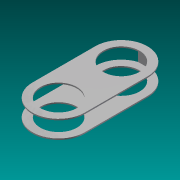
# Autodesk Inventor part: sambungan leaf spring 1
Saved by Autodesk Inventor 2014 SP2 (Build 180246200, 246)
## iProperties
Created: 2019-07-17
Part Number: sambungan leaf spring 1
Material: Steel, Mild
Document SubType Name: Modeling
Designer: USER PC
Density: 7.86 g/cm^3
Appearance: Steel
Author: USER PC
Autodesk Inventor part; units mm, degrees
ref_plane "YZ Plane" through (0, 0, 0) normal (1, 0, 0) x (0, 1, 0)
ref_plane "XZ Plane" through (0, 0, 0) normal (0, 1, 0) x (-1, 0, 0)
ref_plane "XY Plane" through (0, 0, 0) normal (0, 0, 1) x (1, 0, 0)
sketch "Sketch1" plane through (0, 0, 0) normal (0, 0, 1) x (1, 0, 0)
  circle A0 centre (0, 0) radius 35
  circle A1 centre (0, 120) radius 35
  arc A2 (-50, 0) -> (50, 0) centre (0, 0) ccw
  arc A3 (50, 120) -> (-50, 120) centre (0, 120) ccw
  line L0 (-50, 0) -> (-50, 120)
  line L1 (50, 0) -> (50, 120)
  line L2 (0, 35) -> (0, 85)
  dimension "d0" = 70
  dimension "d1" = 70
  dimension "d3" = 15
  dimension "d4" = 15
  dimension "d7" = 50
  constraints: 6 end point, 4 point on circle, 2 centre point, 2 tangent, 2 vertical alignment, 1 coincident, 1 parallel, 4 other
  measures "d7" distance of L2.start L2.end
extrude "Extrusion1" add sketch "Sketch1" along normal blind 35
sketch "Sketch2" plane through (50, 0, 0) normal (1, 0, 0) x (0, 0, -1)
  line L0 (-35, 170) -> (0, 170)
  line L1 (0, 170) -> (0, -50)
  line L2 (0, -50) -> (-35, -50)
  line L3 (-35, -50) -> (-35, 170)
  line L4 (-2.5, -47.5) -> (-2.5, 167.5)
  line L5 (-2.5, 167.5) -> (-32.5, 167.5)
  line L6 (-32.5, 167.5) -> (-32.5, -47.5)
  line L7 (-32.5, -47.5) -> (-32.5, -50)
  line L8 (-2.5, -47.5) -> (-2.5, -50)
  dimension "d8" = 220
  dimension "d9" = 2.5
  constraints: 18 end point, 4 parallel, 2 perpendicular, 2 point on line, 1 collinear, 1 horizontal, 2 other
  measures "d8" distance of L0.end L1.end
  measures "d9" distance between parallel lines of L1 L4
extrude "Extrusion2" cut sketch "Sketch2" against normal blind 300 contours L7 L6 L5 L4 L8 L2
body "Solid1"
